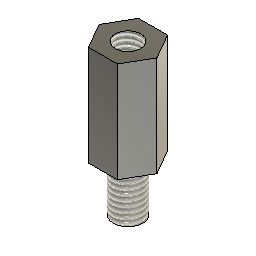
air_quality_sensor (Autodesk Fusion 360 archive; units mm, degrees)
design "dystans 10mm"
Autodesk Fusion 360 part; units mm, degrees
sketch "Sketch1" plane through (0, 0, 0) normal (0, 0, 1) x (1, 0, 0)
  circle A0 centre (0, 0) radius 1.5
  dimension "d1" = 3
  constraint coincident A0.centre origin
  measures "d1" diameter of A0
extrude "Extrude1" add sketch "Sketch1" along normal blind 5
sketch "Sketch2" plane through (0, 0, 5) normal (0, 0, 1) x (-1, 0, 0)
  circle A0 centre (0, 0) radius 1.5
  line L0 (-1.4434, -2.5) -> (1.4434, -2.5)
  line L1 (1.4434, -2.5) -> (2.8868, 0)
  line L2 (2.8868, 0) -> (1.4434, 2.5)
  line L3 (1.4434, 2.5) -> (-1.4434, 2.5)
  line L4 (-1.4434, 2.5) -> (-2.8868, 0)
  line L5 (-2.8868, 0) -> (-1.4434, -2.5)
  dimension "d4" = 2.5
  constraint coincident A0.centre origin
  constraint horizontal L0
  measures "d4" distance of A0.centre L5
extrude "Extrude2" add sketch "Sketch2" along normal blind 12 contours A0 | L0 L1 L2 L3 L4 L5
sketch "Sketch3" plane through (0, 0, 17) normal (0, 0, 1) x (-1, 0, 0)
  line L0 (-2.8868, 0) -> (-1.4434, -2.5)
  line L1 (-1.4434, -2.5) -> (1.4434, -2.5)
  line L2 (1.4434, -2.5) -> (2.8868, 0)
  line L3 (2.8868, 0) -> (1.4434, 2.5)
  line L4 (1.4434, 2.5) -> (-1.4434, 2.5)
  line L5 (-1.4434, 2.5) -> (-2.8868, 0)
  circle A0 centre (0, 0) radius 1.5
  dimension "d7" = 3
  constraint coincident A0.centre origin
  measures "d7" diameter of A0
extrude "Extrude3" cut sketch "Sketch3" against normal blind 10.5 contours A0
thread "Thread1" "ISO Metric profile 3.0 M3x0.5 6H" major diameter 3.086 minor diameter 2.529 pitch 0.5 angle 60 resizes the face on face at (-1.4981, 0.0748, 10)
thread "Thread2" "ISO Metric profile 3.0 M3x0.5 6g" major diameter 2.927 minor diameter 2.3555 pitch 0.5 angle 60 resizes the face on face at (1.4981, 0.0748, 1.6667)
sketch "Sketch4" plane through (0, 0, 17) normal (0, 0, 1) x (-1, 0, 0)
  circle A0 centre (0, 0) radius 1.2645
  line L0 (-2.8868, 0) -> (-1.4434, -2.5)
  line L1 (-1.4434, -2.5) -> (1.4434, -2.5)
  line L2 (1.4434, -2.5) -> (2.8868, 0)
  line L3 (2.8868, 0) -> (1.4434, 2.5)
  line L4 (1.4434, 2.5) -> (-1.4434, 2.5)
  line L5 (-1.4434, 2.5) -> (-2.8868, 0)
  line L6 (12.2401, -7.7834) -> (-13.1427, -7.7834)
  line L7 (-13.1427, -7.7834) -> (-13.1427, 8.3292)
  line L8 (-13.1427, 8.3292) -> (12.2401, 8.3292)
  line L9 (12.2401, 8.3292) -> (12.2401, -7.7834)
  constraint horizontal L6
  constraint vertical L7
  constraint horizontal L8
  constraint vertical L9
extrude "Extrude4" cut sketch "Sketch4" against normal blind 2 contours A0 | L0 L1 L2 L3 L4 L5 | L6 L7 L8 L9

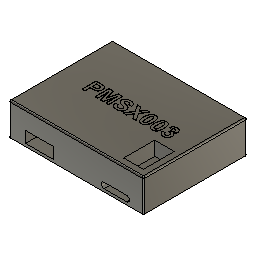
design "PMSX003"
Autodesk Fusion 360 part; units mm, degrees
sketch "Sketch1" plane through (0, 0, 0) normal (0, 0, 1) x (1, 0, 0)
  line L0 (0, 0) -> (48, 0)
  line L1 (48, 0) -> (48, 37)
  line L2 (48, 37) -> (0, 37)
  line L3 (0, 37) -> (0, 0)
  dimension "d1" = 48
  dimension "d2" = 37
  constraint horizontal L0
  constraint vertical L1
  constraint horizontal L2
  constraint vertical L3
  constraint coincident L0.start L3.end
  measures "d1" distance of L0.start L0.end
  measures "d2" distance of L0.start L2.end
extrude "Extrude1" add sketch "Sketch1" along normal blind 12
sketch "Sketch2" plane through (0, 0, 0) normal (0, -1, 0) x (1, 0, 0)
  line L0 (0, 0) -> (48, 0)
  line L1 (48, 0) -> (48, 12)
  line L2 (48, 12) -> (0, 12)
  line L3 (0, 12) -> (0, 0)
  line L4 (6, 1.5) -> (16, 1.5)
  line L5 (16, 1.5) -> (16, 5.5)
  line L6 (16, 5.5) -> (6, 5.5)
  line L7 (6, 5.5) -> (6, 1.5)
  line L8 (33, 3.5) -> (43, 3.5)
  line L9 (43, 3.5) -> (43, 1.5)
  line L10 (43, 1.5) -> (33, 1.5)
  line L11 (33, 1.5) -> (33, 3.5)
  dimension "d5" = 1.5
  dimension "d6" = 1.5
  dimension "d7" = 10
  dimension "d8" = 2
  dimension "d9" = 5
  dimension "d10" = 10
  dimension "d11" = 4
  dimension "d12" = 6
  constraint horizontal L4
  constraint vertical L5
  constraint horizontal L6
  constraint vertical L7
  constraint horizontal L8
  constraint vertical L9
  constraint horizontal L10
  constraint vertical L11
  measures "d5" distance of L0 L4
  measures "d6" distance of L0 L10
  measures "d7" distance of L8.start L8.end
  measures "d8" distance of L8.end L9.end
  measures "d9" distance of L1 L9
  measures "d10" distance of L5.end L6.end
  measures "d11" distance of L4.start L6.end
  measures "d12" distance of L3 L7
extrude "Extrude2" cut sketch "Sketch2" against normal blind 10 contours L4 L5 L6 L7 | L8 L9 L10 L11
fillet "Fillet1" radius 1 4 edges at (33, 5, 3.5) (33, 5, 1.5) (43, 5, 3.5) (43, 5, 1.5)
sketch "Sketch3" plane through (0, 0, 12) normal (0, 0, 1) x (-1, 0, 0)
  line L0 (0, -37) -> (0, 0)
  line L1 (0, 0) -> (-48, 0)
  line L2 (-48, 0) -> (-48, -37)
  line L3 (-48, -37) -> (0, -37)
  line L4 (-38.5, -13.5) -> (-45.5, -13.5)
  line L5 (-45.5, -13.5) -> (-45.5, -2.5)
  line L6 (-45.5, -2.5) -> (-38.5, -2.5)
  line L7 (-38.5, -2.5) -> (-38.5, -13.5)
  dimension "d17" = 7
  dimension "d18" = 11
  dimension "d19" = 2.5
  dimension "d20" = 2.5
  constraint horizontal L4
  constraint vertical L5
  constraint horizontal L6
  constraint vertical L7
  measures "d17" distance of L5.end L6.end
  measures "d18" distance of L4.end L5.end
  measures "d19" distance of L1 L6
  measures "d20" distance of L2 L5
extrude "Extrude3" cut sketch "Sketch3" against normal blind 5 contours L4 L5 L6 L7
sketch "Sketch4" plane through (0, 0, 12) normal (0, 0, 1) x (-1, 0, 0)
  line L0 (-45.5, -13.5) -> (-45.5, -2.5)
  line L1 (-45.5, -2.5) -> (-38.5, -2.5)
  line L2 (-38.5, -2.5) -> (-38.5, -13.5)
  line L3 (-38.5, -13.5) -> (-45.5, -13.5)
  line L4 (0, -37) -> (0, 0)
  line L5 (0, 0) -> (-48, 0)
  line L6 (-48, 0) -> (-48, -37)
  line L7 (-48, -37) -> (0, -37)
  line L8 (-9.7834, -15.2708) -> (-37.5329, -15.2708) construction
  line L9 (-37.5329, -15.2708) -> (-37.5329, -21.3337) construction
  line L10 (-37.5329, -21.3337) -> (-9.7834, -21.3337) construction
  line L11 (-9.7834, -21.3337) -> (-9.7834, -15.2708) construction
  text T0 "PMSX003" font "Arial" height 5 bold align left top in box 27.7495 x 6.0629 at (-9.7834, -15.2708) x (-1, 0) y (0, -1) spacing 1 kerned
extrude "Extrude4" cut sketch "Sketch4" against normal blind 0.1 text T0
fillet "Fillet2" radius 0.5 12 edges at (0, 18.5, 0) (0, 18.5, 12) (24, 0, 12) (0, 0, 6) (0, 37, 6) (24, 37, 12) (24, 37, 0) (48, 37, 6) (48, 18.5, 12) (48, 18.5, 0) (48, 0, 6) (24, 0, 0)
